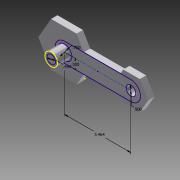
# Autodesk Inventor part: Frame
Saved by Autodesk Inventor 2018 (Build 220112000, 112)
## iProperties
Created: 2018-01-20
Part Number: Frame
Material: ABS Plastic
Document SubType Name: Modeling
Designer: Rus
Density: 1.06 g/cm^3
Appearance: Smooth - White
Author: Rus
Autodesk Inventor part; units mm, degrees
ref_plane "YZ Plane" through (0, 0, 0) normal (1, 0, 0) x (0, 1, 0)
ref_plane "XZ Plane" through (0, 0, 0) normal (0, 1, 0) x (-1, 0, 0)
ref_plane "XY Plane" through (0, 0, 0) normal (0, 0, 1) x (1, 0, 0)
sketch "Sketch1" plane through (0, 0, 0) normal (0, 0, 1) x (1, 0, 0)
  circle A0 centre (-43.9941, 0) radius 9.525
  circle A1 centre (43.9941, 0) radius 6.35
  line L0 (43.9941, 0) -> (-43.9941, 0) construction
  line L1 (43.9941, 12.7) -> (-43.9941, 12.7)
  line L2 (-43.9941, -12.7) -> (43.9941, -12.7)
  arc A2 (43.9941, -12.7) -> (43.9941, 12.7) centre (43.9941, 0) ccw
  arc A3 (-43.9941, 12.7) -> (-43.9941, -12.7) centre (-43.9941, 0) ccw
  point P0 (0, 0)
  point P1 (0, 0)
  dimension "d10" = 12.7
  dimension "d11" = 19.05
  dimension "d12" = 87.9881
  dimension "d13" = 12.7
  constraints: 8 end point, 4 centre point, 4 point on circle, 4 tangent, 1 coincident, 1 horizontal, 1 midpoint, 1 parallel
  measures "d10" diameter of A1
  measures "d11" diameter of A0
  measures "d12" distance of L0.start L0.end
  measures "d13" distance of L2.start L0.end
sketch "Sketch3" plane through (0, 0, 0) normal (0, 0, 1) x (1, 0, 0)
  line L0 (-44.9008, 0) -> (44.9008, 0) construction
  line L1 (-44.9008, -12.7) -> (44.9008, -12.7)
  line L2 (44.9008, 12.7) -> (-44.9008, 12.7)
  arc A0 (-44.9008, 12.7) -> (-44.9008, -12.7) centre (-44.9008, 0) ccw
  arc A1 (44.9008, -12.7) -> (44.9008, 12.7) centre (44.9008, 0) ccw
  circle A2 centre (-44.9008, 0) radius 6.35
  point P0 (0, 0)
  dimension "d23" = 44.9008
  dimension "d24" = 25.4
  dimension "d25" = 12.7
  constraints: 8 end point, 4 point on circle, 4 tangent, 3 centre point, 1 coincident, 1 horizontal, 1 midpoint, 1 parallel
  measures "d23" distance of point (0, 0) L0.end
  measures "d24" distance between parallel lines of L1 L2
  measures "d25" diameter of A2
extrude "Extrusion4" add sketch "Sketch3" against normal blind 8.4667
sketch "Sketch4" plane through (0, 0, -8.4667) normal (0, 0, -1) x (-1, 0, 0)
  circle A0 centre (-44.9008, 0) radius 6.35
  arc A1 (-44.9008, 12.7) -> (-44.9008, -12.7) centre (-44.9008, 0) ccw projected
  point P0 (0, 0)
  dimension "d28" = 12.7
  constraints: 1 centre point, 1 coincident
  measures "d28" diameter of A0
extrude "Extrusion5" cut sketch "Sketch4" against normal through all
sketch "Sketch5" plane through (0, 0, -8.4667) normal (0, 0, -1) x (-1, 0, 0)
  circle A0 centre (44.9008, 0) radius 6.35 projected
  line L0 (61.8342, 29.3294) -> (78.7675, 0)
  line L1 (78.7675, 0) -> (61.8342, -29.3294)
  line L2 (61.8342, -29.3294) -> (27.9675, -29.3294)
  line L3 (27.9675, -29.3294) -> (11.0342, 0)
  line L4 (11.0342, 0) -> (27.9675, 29.3294)
  line L5 (27.9675, 29.3294) -> (61.8342, 29.3294)
  line L6 (-44.9008, 12.7) -> (44.9008, 12.7) projected
  point P0 (0, 0)
  dimension "d31" = 33.8667
  constraints: 12 end point, 2 coincident, 1 parallel, 13 other
  measures "d31" distance of L4.end L0.start
extrude "Extrusion6" add sketch "Sketch5" against normal up to surface (8.4667 mm away)
sketch "Sketch7" plane through (0, 0, -8.4667) normal (0, 0, -1) x (-1, 0, 0)
  circle A0 centre (-44.9008, 0) radius 6.35 projected
  circle A1 centre (-44.9008, 0) radius 12.7
  line L0 (-44.9008, -12.7) -> (18.3665, -12.7) projected
  line L1 (-66.8979, 0) -> (-55.8994, 19.05)
  line L2 (-55.8994, 19.05) -> (-33.9023, 19.05)
  line L3 (-33.9023, 19.05) -> (-22.9038, 0)
  line L4 (-22.9038, 0) -> (-33.9023, -19.05)
  line L5 (-33.9023, -19.05) -> (-55.8994, -19.05)
  line L6 (-55.8994, -19.05) -> (-66.8979, 0)
  point P0 (0, 0)
  point P1 (5.3062, -12.7)
  dimension "d48" = 38.1
  constraints: 13 end point, 2 coincident, 1 centre point, 1 horizontal, 1 tangent, 13 other
  measures "d48" distance between parallel lines of L5 L2
extrude "Extrusion8" add sketch "Sketch7" against normal up to surface (8.4667 mm away) contours L1 L2 L3 L4 L5 L6
sketch "Sketch12" plane through (0, 0, -8.4667) normal (0, 0, -1) x (-1, 0, 0)
  circle A0 centre (44.9008, 0) radius 6.35 projected
  circle A1 centre (44.9008, 0) radius 8.4667
  point P0 (0, 0)
  dimension "d73" = 16.9333
  constraints: 1 centre point, 1 coincident
  measures "d73" diameter of A1
extrude "Extrusion12" add sketch "Sketch12" against normal blind 25.4 contours A0 | A1
sketch "Sketch13" plane through (-44.9008, 0, 16.9333) normal (0, 0, 1) x (1, 0, 0)
  circle A0 centre (0, 0) radius 8.4667 projected
  circle A1 centre (0, 0) radius 8.4667 projected
  circle A2 centre (0, 0) radius 5.6444
  point P0 (44.9008, 0)
  dimension "d76" = 11.2889
  constraints: 1 centre point, 1 coincident
  measures "d76" diameter of A2
extrude "Extrusion13" cut sketch "Sketch13" against normal blind 11.2889 draft -10 contours A2
sketch "Sketch14" plane through (0, 0, -8.4667) normal (0, 0, -1) x (-1, 0, 0)
  circle A0 centre (-44.9008, 0) radius 6.35 projected
  circle A1 centre (-44.9008, 0) radius 6.35
  point P0 (0, 0)
  dimension "d79" = 12.7
  constraints: 1 centre point, 1 coincident
  measures "d79" diameter of A1
extrude "Extrusion14" add sketch "Sketch14" against normal blind 25.4
sketch "Sketch15" plane through (44.9008, 0, 16.9333) normal (0, 0, 1) x (1, 0, 0)
  circle A0 centre (0, 0) radius 6.35 projected
  circle A1 centre (0, 0) radius 4.2333
  point P0 (-44.9008, 0)
  dimension "d82" = 8.4667
  constraints: 1 centre point, 1 coincident
  measures "d82" diameter of A1
extrude "Extrusion15" cut sketch "Sketch15" against normal blind 11.2889 draft -10 contours A1
body "Solid2"
